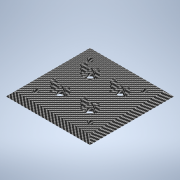
# Autodesk Inventor part: Base Plate
Saved by Autodesk Inventor 2021.1 (Build 251245010, 245A)
## iProperties
Created: 2020-11-23
Part Number: Base Plate
Material: CFRP
Document SubType Name: Modeling
Designer: elizh
Density: 1.43 g/cm^3
Appearance: Carbon Fiber
Author: elizh
Autodesk Inventor part; units mm, degrees
ref_plane "YZ Plane" through (0, 0, 0) normal (1, 0, 0) x (0, 1, 0)
ref_plane "XZ Plane" through (0, 0, 0) normal (0, 1, 0) x (-1, 0, 0)
ref_plane "XY Plane" through (0, 0, 0) normal (0, 0, 1) x (1, 0, 0)
sketch "Sketch1" plane through (0, 0, 0) normal (0, 1, 0) x (-1, 0, 0)
  line L0 (45, 45) -> (-45, 45)
  line L1 (-45, 45) -> (-45, -45)
  line L2 (-45, -45) -> (45, -45)
  line L3 (45, -45) -> (45, 45)
  line L4 (0, 0) -> (55.2623, 0) construction
  line L5 (0, 0) -> (0, -72.148) construction
  dimension "d0" = 90
  constraints: 12 end point, 2 horizontal, 2 parallel, 2 perpendicular, 1 vertical, 2 other
  measures "d0" distance of L2.end L0.start
extrude "Extrusion1" add sketch "Sketch1" along normal blind 5
chamfer "Chamfer2" distance 5 angle 45 4 edges at (-45, 5, 0) (0, 5, -45) (45, 5, 0) (0, 5, 45)
sketch "Sketch5" plane through (0, 5, 0) normal (0, 1, 0) x (1, 0, 0)
  line L0 (-22, -22) -> (-10, -22)
  line L1 (-10, -22) -> (-10, -10)
  line L2 (-10, -10) -> (-22, -10)
  line L3 (-22, -10) -> (-22, -22)
  line L4 (0, 0) -> (-17.5876, 0) construction
  line L5 (0, 0) -> (0, 27.0417) construction
  line L6 (22, -22) -> (10, -22)
  line L7 (10, -22) -> (10, -10)
  line L8 (10, -10) -> (22, -10)
  line L9 (22, -10) -> (22, -22)
  line L10 (-22, 22) -> (-10, 22)
  line L11 (-10, 22) -> (-10, 10)
  line L12 (-10, 10) -> (-22, 10)
  line L13 (-22, 10) -> (-22, 22)
  line L14 (22, 22) -> (10, 22)
  line L15 (10, 22) -> (10, 10)
  line L16 (10, 10) -> (22, 10)
  line L17 (22, 10) -> (22, 22)
  dimension "d13" = 12
  dimension "d14" = 10
  dimension "d15" = 10
  constraints: 36 end point, 12 symmetric about line, 2 horizontal, 2 parallel, 2 perpendicular, 1 vertical
  measures "d13" distance of L2.end L0.start
  measures "d14" distance between parallel lines of L4 L2
  measures "d15" distance between parallel lines of L5 L1
extrude "Extrusion3" cut sketch "Sketch5" against normal blind 2
sketch "Sketch6" plane through (0, 3, 0) normal (0, 1, 0) x (1, 0, 0)
  line L0 (-10, -10) -> (-10, -22) construction
  line L1 (-22, -10) -> (-10, -10) construction
  line L2 (-22, -22) -> (-22, -10) construction
  line L3 (-10, -22) -> (-22, -22) construction
  circle A0 centre (-16, -16.4511) radius 6 construction
  line L4 (-22, -22) -> (-22, -10) construction
  line L5 (-10, -10) -> (-10, -22) construction
  circle A1 centre (-16, -16.4511) radius 3.5
  line L6 (0, 0) -> (0, 11.1896) construction
  line L7 (0, 0) -> (9.9174, 0) construction
  circle A2 centre (16, -16.4511) radius 3.5
  circle A3 centre (-16, 16.4511) radius 3.5
  circle A4 centre (16, 16.4511) radius 3.5
  dimension "d18" = 7
  constraints: 5 centre point, 4 end point, 3 symmetric about line, 2 tangent, 1 concentric, 1 horizontal, 1 vertical, 3 other
  measures "d18" diameter of A1
extrude "Extrusion4" cut sketch "Sketch6" against normal through all
sketch "Sketch7" plane through (0, 5, 0) normal (0, 1, 0) x (1, 0, 0)
  line L0 (-10, -22) -> (-22, -22) construction
  line L1 (-22, -22) -> (-22, -10) construction
  line L2 (-22, -10) -> (-10, -10) construction
  line L3 (-10, -10) -> (-10, -22) construction
  line L4 (-22, -22) -> (-22, -10) construction
  line L5 (-22, -10) -> (-10, -10) construction
  line L6 (-10, -10) -> (-10, -22) construction
  line L7 (-22, -18.5) -> (-24, -18.5)
  line L8 (-24, -18.5) -> (-24, -13.5)
  line L9 (-24, -13.5) -> (-22, -13.5)
  line L10 (-22, -13.5) -> (-22, -18.5)
  line L11 (-10, -18.5) -> (-8, -18.5)
  line L12 (-8, -18.5) -> (-8, -13.5)
  line L13 (-8, -13.5) -> (-10, -13.5)
  line L14 (-10, -13.5) -> (-10, -18.5)
  line L15 (0, 0) -> (0, 13.7984) construction
  line L16 (0, 0) -> (13.8791, 0) construction
  line L17 (22, -18.5) -> (24, -18.5)
  line L18 (24, -18.5) -> (24, -13.5)
  line L19 (24, -13.5) -> (22, -13.5)
  line L20 (22, -13.5) -> (22, -18.5)
  line L21 (10, -18.5) -> (8, -18.5)
  line L22 (8, -18.5) -> (8, -13.5)
  line L23 (8, -13.5) -> (10, -13.5)
  line L24 (10, -13.5) -> (10, -18.5)
  line L25 (-22, 18.5) -> (-24, 18.5)
  line L26 (-24, 18.5) -> (-24, 13.5)
  line L27 (-24, 13.5) -> (-22, 13.5)
  line L28 (-22, 13.5) -> (-22, 18.5)
  line L29 (-10, 18.5) -> (-8, 18.5)
  line L30 (-8, 18.5) -> (-8, 13.5)
  line L31 (-8, 13.5) -> (-10, 13.5)
  line L32 (-10, 13.5) -> (-10, 18.5)
  line L33 (8, 13.5) -> (10, 13.5)
  line L34 (10, 18.5) -> (8, 18.5)
  line L35 (8, 18.5) -> (8, 13.5)
  line L36 (10, 13.5) -> (10, 18.5)
  line L37 (24, 13.5) -> (22, 13.5)
  line L38 (22, 13.5) -> (22, 18.5)
  line L39 (24, 18.5) -> (24, 13.5)
  line L40 (22, 18.5) -> (24, 18.5)
  dimension "d22" = 3.5
  dimension "d23" = 3.5
  dimension "d24" = 2
  dimension "d25" = 2
  constraints: 68 end point, 24 symmetric about line, 10 point on line, 4 parallel, 3 horizontal, 2 perpendicular, 1 vertical
  measures "d22" distance between parallel lines of L7 L0
  measures "d23" distance between parallel lines of L2 L9
  measures "d24" distance between parallel lines of L1 L8
  measures "d25" distance between parallel lines of L3 L12
extrude "Extrusion5" add sketch "Sketch7" along normal blind 4
sketch "Sketch8" plane through (0, 9, 0) normal (0, 1, 0) x (1, 0, 0)
  line L0 (-22, -13.5) -> (-24, -13.5) projected
  line L1 (-24, -13.5) -> (-24, -18.5) projected
  line L2 (-24, -18.5) -> (-22, -18.5) projected
  line L3 (-22, -18.5) -> (-22, -13.5) construction
  line L4 (-8, -18.5) -> (-8, -13.5) projected
  line L5 (-8, -13.5) -> (-10, -13.5) projected
  line L6 (-10, -13.5) -> (-10, -18.5) construction
  line L7 (-10, -18.5) -> (-8, -18.5) projected
  line L8 (-22, -18.5) -> (-21, -18.5)
  line L9 (-21, -18.5) -> (-21, -13.5)
  line L10 (-21, -13.5) -> (-22, -13.5)
  line L11 (-22, -13.5) -> (-22, -18.5) construction
  line L12 (-10, -13.5) -> (-10, -18.5) construction
  line L13 (-10, -18.5) -> (-11, -18.5)
  line L14 (-11, -18.5) -> (-11, -13.5)
  line L15 (-11, -13.5) -> (-9.9096, -13.5)
  line L16 (0, 0) -> (0, 11.7136) construction
  line L17 (0, 0) -> (17.2625, 0) construction
  line L18 (22, -13.5) -> (24, -13.5)
  line L19 (24, -13.5) -> (24, -18.5)
  line L20 (24, -18.5) -> (22, -18.5)
  line L21 (22, -18.5) -> (22, -13.5) construction
  line L22 (8, -18.5) -> (8, -13.5)
  line L23 (8, -13.5) -> (10, -13.5)
  line L24 (10, -13.5) -> (10, -18.5) construction
  line L25 (10, -18.5) -> (8, -18.5)
  line L26 (22, -18.5) -> (21, -18.5)
  line L27 (21, -18.5) -> (21, -13.5)
  line L28 (21, -13.5) -> (22, -13.5)
  line L29 (22, -13.5) -> (22, -18.5) construction
  line L30 (10, -13.5) -> (10, -18.5) construction
  line L31 (10, -18.5) -> (11, -18.5)
  line L32 (11, -18.5) -> (11, -13.5)
  line L33 (11, -13.5) -> (9.9096, -13.5)
  line L34 (-22, 13.5) -> (-24, 13.5)
  line L35 (-24, 13.5) -> (-24, 18.5)
  line L36 (-24, 18.5) -> (-22, 18.5)
  line L37 (-22, 18.5) -> (-22, 13.5) construction
  line L38 (-8, 18.5) -> (-8, 13.5)
  line L39 (-8, 13.5) -> (-10, 13.5)
  line L40 (-10, 13.5) -> (-10, 18.5) construction
  line L41 (-10, 18.5) -> (-8, 18.5)
  line L42 (-22, 18.5) -> (-21, 18.5)
  line L43 (-21, 18.5) -> (-21, 13.5)
  line L44 (-21, 13.5) -> (-22, 13.5)
  line L45 (-22, 13.5) -> (-22, 18.5) construction
  line L46 (-10, 13.5) -> (-10, 18.5) construction
  line L47 (-10, 18.5) -> (-11, 18.5)
  line L48 (-11, 18.5) -> (-11, 13.5)
  line L49 (-11, 13.5) -> (-9.9096, 13.5)
  line L50 (8, 13.5) -> (10, 13.5)
  line L51 (11, 13.5) -> (9.9096, 13.5)
  line L52 (8, 18.5) -> (8, 13.5)
  line L53 (10, 18.5) -> (8, 18.5)
  line L54 (10, 13.5) -> (10, 18.5) construction
  line L55 (10, 13.5) -> (10, 18.5) construction
  line L56 (11, 18.5) -> (11, 13.5)
  line L57 (21, 13.5) -> (22, 13.5)
  line L58 (22, 13.5) -> (24, 13.5)
  line L59 (21, 18.5) -> (21, 13.5)
  line L60 (22, 18.5) -> (22, 13.5) construction
  line L61 (22, 18.5) -> (21, 18.5)
  line L62 (22, 13.5) -> (22, 18.5) construction
  line L63 (24, 13.5) -> (24, 18.5)
  line L64 (24, 18.5) -> (22, 18.5)
  line L65 (10, 18.5) -> (11, 18.5)
  dimension "d28" = 1
  dimension "d29" = 1
  constraints: 114 end point, 42 symmetric about line, 4 point on line, 3 horizontal, 3 parallel, 2 perpendicular, 1 collinear, 1 vertical
  measures "d28" distance between parallel lines of L9 L3
  measures "d29" distance between parallel lines of L14 L6
extrude "Extrusion6" add sketch "Sketch8" along normal blind 3
chamfer "Chamfer3" distance 1 distance2 3 1 edges at (-21, 12, 16) measured on face at (-22, 12, 16.8333)
chamfer "Chamfer4" distance 1 distance2 3 1 edges at (-11, 12, 16) measured on face at (-10, 12, 16.8333)
chamfer "Chamfer5" distance 1 distance2 3 1 edges at (11, 12, 16) measured on face at (10, 12, 16.8333)
chamfer "Chamfer6" distance 1 distance2 3 1 edges at (21, 12, 16) measured on face at (22, 12, 16.8333)
chamfer "Chamfer7" distance 1 distance2 3 1 edges at (-21, 12, -16) measured on face at (-22, 12, -16.8333)
chamfer "Chamfer8" distance 1 distance2 3 1 edges at (-11, 12, -16) measured on face at (-10, 12, -16.8333)
chamfer "Chamfer9" distance 1 distance2 3 1 edges at (11, 12, -16) measured on face at (10, 12, -16.8333)
chamfer "Chamfer10" distance 1 distance2 3 1 edges at (21, 12, -16) measured on face at (22, 12, -16.8333)
sketch "Sketch10" plane through (0, 5, 0) normal (0, 1, 0) x (1, 0, 0)
  line L0 (0, 0) -> (-26.6141, 0) construction
  line L1 (0, 0) -> (0, 28.7963) construction
  circle A0 centre (-29, -29) radius 2.75
  circle A1 centre (-29, 29) radius 2.75
  circle A2 centre (29, -29) radius 2.75
  circle A3 centre (29, 29) radius 2.75
  point P0 (26.6141, 0)
  dimension "d56" = 29
  dimension "d57" = 5.5
  dimension "d58" = 29
  constraints: 4 centre point, 4 end point, 4 symmetric about line, 1 horizontal, 1 vertical, 3 other
  measures "d56" distance from line of L0 A0.centre
  measures "d57" diameter of A0
  measures "d58" distance from line of L1 A0.centre
extrude "Extrusion7" cut sketch "Sketch10" against normal blind 4
equation "\"d22\" = d23"
equation "\"d25\" = d24"
equation "\"d58\" = d56"
body "Solid1"
